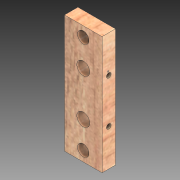
# Autodesk Inventor part: 12112_Proximal Roller Plate_V1
Saved by Autodesk Inventor 2020 (Build 240168000, 168)
## iProperties
Created: 2019-09-30
Part Number: 12112_Proximal Roller Plate_V1
Material: Wood (Birch)
Document SubType Name: Modeling
Designer: MPI
Density: 0.55 g/cm^3
Appearance: Birch - Natural Polished
Author: MPI
Autodesk Inventor part; units mm, degrees
ref_plane "YZ Plane" through (0, 0, 0) normal (1, 0, 0) x (0, 1, 0)
ref_plane "XZ Plane" through (0, 0, 0) normal (0, 1, 0) x (-1, 0, 0)
ref_plane "XY Plane" through (0, 0, 0) normal (0, 0, 1) x (1, 0, 0)
sketch "Sketch1" plane through (0, 0, 0) normal (0, 0, 1) x (1, 0, 0)
  line L0 (-14, 44) -> (14, 44)
  line L1 (14, 44) -> (14, -44)
  line L2 (14, -44) -> (-14, -44)
  line L3 (-14, -44) -> (-14, 44)
  circle A0 centre (0, 16.5) radius 4.8
  circle A1 centre (0, -16.5) radius 4.8
  circle A2 centre (0, 36.5) radius 4.25
  circle A3 centre (0, -36.5) radius 4.25
  point P0 (0, 0)
  dimension "d0" = 28
  dimension "d2" = 9.6
  dimension "d3" = 9.6
  dimension "d8" = 8.5
  dimension "d9" = 8.5
  dimension "d11" = 20
  dimension "d12" = 20
  dimension "d37" = 44
  dimension "d38" = 44
  dimension "d45" = 33
  constraints: 8 end point, 4 centre point, 2 parallel, 1 horizontal, 1 perpendicular
  measures "d0" distance of L0.start L0.end
  measures "d2" diameter of A0
  measures "d3" diameter of A1
  measures "d8" diameter of A2
  measures "d9" diameter of A3
  measures "d11" distance of A0.centre A2.centre
  measures "d12" distance of A3.centre A1.centre
  measures "d37" distance from line of point (0, 0) L0
  measures "d38" distance from line of L2 point (0, 0)
  measures "d45" distance of A1.centre A0.centre
extrude "Extrusion1" add sketch "Sketch1" along normal blind 10
sketch "Sketch2" plane through (14, -44, 0) normal (1, 0, 0) x (0, 0, -1)
  circle A0 centre (-5, 60.5) radius 1.725
  circle A1 centre (-5, 27.5) radius 1.725
  line L0 (-10, 0) -> (-10, 88) projected
  point P0 (0, 44)
  dimension "d23" = 3.45
  dimension "d24" = 3.45
  dimension "d25" = 16.5
  dimension "d26" = 16.5
  dimension "d27" = 5
  dimension "d28" = 5
  constraints: 2 centre point
  measures "d23" diameter of A0
  measures "d24" diameter of A1
  measures "d25" vertical distance of point (0, 44) A0.centre
  measures "d26" vertical distance of A1.centre point (0, 44)
  measures "d27" distance from line of L0 A0.centre
  measures "d28" distance from line of L0 A1.centre
extrude "Extrusion2" cut sketch "Sketch2" against normal blind 15
body "Solid1"
